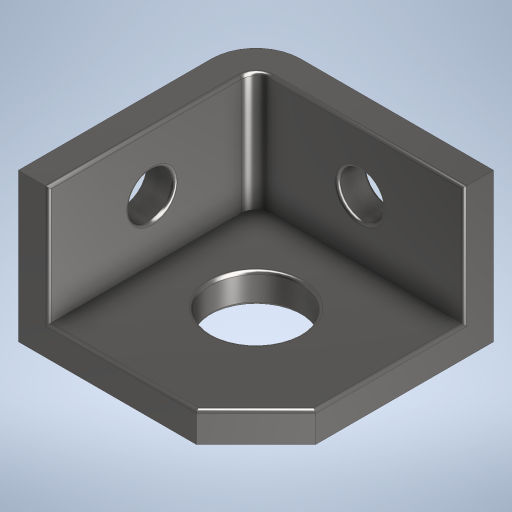
# Autodesk Inventor part: Basics
Saved by Autodesk Inventor 2024.3 (Build 283343000, 343)
## iProperties
Created: 2026-06-11
Part Number: Basics
Material: Steel, Cast
Document SubType Name: Modeling
Designer: scott
Density: 7.85 g/cm^3
Appearance: Semi-Polished
Author: scott
Autodesk Inventor part; units mm, degrees
ref_plane "YZ Plane" through (0, 0, 0) normal (1, 0, 0) x (0, 1, 0)
ref_plane "XZ Plane" through (0, 0, 0) normal (0, 1, 0) x (-1, 0, 0)
ref_plane "XY Plane" through (0, 0, 0) normal (0, 0, 1) x (1, 0, 0)
sketch "Sketch1" plane through (0, 0, 0) normal (0, 1, 0) x (-1, 0, 0)
  line L0 (0, 0) -> (20.32, 0)
  line L1 (20.32, 0) -> (20.32, -20.32)
  line L2 (20.32, -20.32) -> (0, -20.32)
  line L3 (0, -20.32) -> (0, 0)
  circle A0 centre (10.16, -10.16) radius 3.81
  line L4 (5.08, 0) -> (11.3037, 0) construction
  line L5 (5.08, 0) -> (0, -5.08)
  line L6 (5.08, 0) -> (12.2642, 0) construction
  dimension "d0" = 20.32
  dimension "d1" = 20.32
  dimension "d2" = 7.62
  dimension "d3" = 10.16
  dimension "d4" = 10.16
  dimension "d6" = 135
  dimension "d7" = 5.08
  dimension "d8" = 5.08
  constraints: 14 end point, 3 horizontal, 2 parallel, 2 point on line, 1 centre point, 1 equal length, 1 perpendicular
  measures "d0" distance of L1.end L2.end
  measures "d1" distance of L0.end L1.end
  measures "d2" diameter of A0
  measures "d3" distance from line of L1 A0.centre
  measures "d4" distance from line of L2 A0.centre
  measures "d6" angle of L5 L6
  measures "d7" distance from line of L3 L4.start
  measures "d8" distance of L0.start L5.end
extrude "Extrusion1" add sketch "Sketch1" along normal blind 2.54 contours L0 L1 L2 L3 L5
sketch "Sketch2" plane through (0, 2.54, 0) normal (0, 1, 0) x (1, 0, 0)
  line L0 (-20.32, 20.32) -> (-20.32, 0) projected
  line L1 (0, 20.32) -> (-20.32, 20.32) projected
  line L2 (-20.32, 0) -> (-17.78, 0)
  line L3 (-17.78, 0) -> (-17.78, 20.32)
  line L4 (-17.78, 20.32) -> (-20.32, 20.32)
  line L5 (-20.32, 20.32) -> (-20.32, 0)
  line L6 (0, 5.08) -> (0, 20.32) projected
  line L7 (0, 20.32) -> (-20.32, 20.32)
  line L8 (-20.32, 20.32) -> (-20.32, 17.78)
  line L9 (-20.32, 17.78) -> (0, 17.78)
  line L10 (0, 17.78) -> (0, 20.32)
  point P0 (0, 0)
  point P1 (-17.78, 17.78)
  dimension "d11" = 2.54
  dimension "d12" = 2.54
  constraints: 16 end point, 4 parallel, 2 horizontal, 2 perpendicular, 2 point on line
  measures "d11" distance of L4.end L3.end
  measures "d12" distance of L8.end L7.end
extrude "Extrusion2" add sketch "Sketch2" along normal blind 10.16
fillet "Fillet1" radius 1.27 1 edges at (-17.78, 7.62, -17.78)
fillet "Fillet2" radius 3.81 1 edges at (-20.32, 6.35, -20.32)
sketch "Sketch3" plane through (-17.78, 2.54, 0) normal (1, 0, 0) x (0, 0, -1)
  circle A0 centre (8.89, 5.08) radius 1.905
  line L0 (0, 10.16) -> (16.51, 10.16) projected
  line L1 (0, 0) -> (0, 10.16) projected
  point P0 (0, -2.54)
  dimension "d17" = 3.81
  dimension "d18" = 5.08
  dimension "d19" = 8.89
  constraints: 1 centre point
  measures "d17" diameter of A0
  measures "d18" distance from line of L0 A0.centre
  measures "d19" distance from line of L1 A0.centre
extrude "Extrusion3" cut sketch "Sketch3" against normal blind 10.16
sketch "Sketch4" plane through (0, 2.54, -17.78) normal (0, 0, 1) x (1, 0, 0)
  circle A0 centre (-8.89, 5.08) radius 1.905
  line L0 (-16.51, 10.16) -> (0, 10.16) projected
  line L1 (0, 0) -> (0, 10.16) projected
  point P0 (0, -2.54)
  point P1 (0, 5.08)
  dimension "d22" = 3.81
  dimension "d23" = 5.08
  dimension "d24" = 8.89
  constraints: 1 centre point, 1 midpoint
  measures "d22" diameter of A0
  measures "d23" distance from line of L0 A0.centre
  measures "d24" distance of point (0, 5.08) A0.centre
extrude "Extrusion4" cut sketch "Sketch4" against normal blind 10.16
fillet "Fillet3" radius 0.254 14 edges at (-17.408, 12.7, -17.408) (-8.255, 12.7, -17.78) (-17.78, 12.7, -8.255) (0, 7.62, -17.78) (0, 2.54, -11.43) (-2.54, 2.54, -2.54) (-11.43, 2.54, 0) (-17.78, 7.62, 0) (-10.795, 7.62, -17.78) (-17.78, 7.62, -6.985) (-10.795, 7.62, -20.32) (-20.32, 7.62, -6.985) (-6.35, 0, -10.16) (-6.35, 2.54, -10.16)
body "Solid1"
